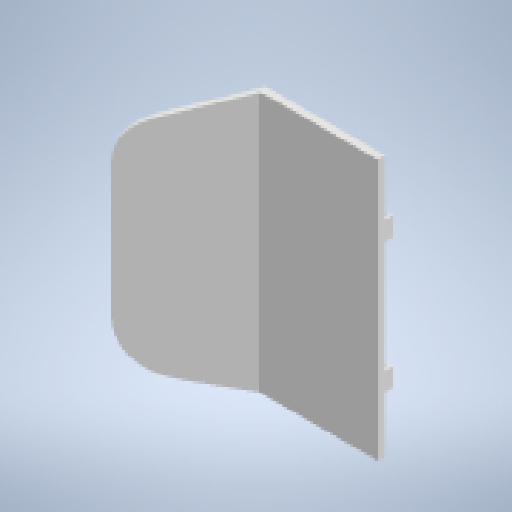
# Autodesk Inventor part: case
Saved by Autodesk Inventor 2025 (Build 290162000, 162)
## iProperties
Created: 2025-08-16
Part Number: case
Material: Generic
Document SubType Name: Modeling
Designer: naka6
Density: 1 g/cm^3
Appearance: Default
Author: naka6
Autodesk Inventor part; units mm, degrees
ref_plane "YZ Plane" through (0, 0, 0) normal (1, 0, 0) x (0, 1, 0)
ref_plane "XZ Plane" through (0, 0, 0) normal (0, 1, 0) x (-1, 0, 0)
ref_plane "XY Plane" through (0, 0, 0) normal (0, 0, 1) x (1, 0, 0)
sketch "スケッチ1" plane through (0, 0, 0) normal (0, 0, 1) x (1, 0, 0)
  line L0 (0, 0) -> (-32, 0)
  line L1 (-32, 0) -> (-32, -70)
  line L2 (-32, -70) -> (0, -70)
  line L3 (0, -70) -> (0, 0)
  dimension "d0" = 32
  dimension "d1" = 70
  constraints: 8 end point, 2 parallel, 1 horizontal, 1 perpendicular
  measures "d0" distance of L0.start L0.end
  measures "d1" distance of L2.end L0.start
extrude "押し出し1" add sketch "スケッチ1" along normal blind 2
sketch "スケッチ2" plane through (-32, -70, 0) normal (0, -1, 0) x (1, 0, 0)
  line L0 (0, 0) -> (32, 0) projected
  line L1 (32, 0) -> (32, 2) projected
  line L2 (0, 2) -> (32, 2) projected
  line L3 (0, 0) -> (0, 2) projected
  line L4 (0, 0) -> (-25.9808, 15)
  line L5 (-25.9808, 15) -> (-25.1147, 16.5)
  line L6 (-25.1147, 16.5) -> (0, 2)
  point P0 (32, 0)
  dimension "d4" = 30
  dimension "d5" = 150
  constraints: 6 end point, 2 perpendicular
  measures "d4" distance of L0.start L4.end
  measures "d5" angle of L2 L6
extrude "押し出し2" add sketch "スケッチ2" against normal blind 70 contours L4 L5 L6 L3
sketch "スケッチ3" plane through (0, 0, 0) normal (0, 0, -1) x (-1, 0, 0)
  line L0 (0, 0) -> (32, 0) projected
  line L1 (32, 0) -> (57.9808, -12.115)
  line L2 (32, 0) -> (57.9808, 0) projected
  line L3 (57.9808, -70) -> (57.9808, 0) projected
  dimension "d8" = 25
  constraints: 2 end point, 1 point on line
  measures "d8" angle of L2 L1
extrude "押し出し3" cut sketch "スケッチ3" against normal blind 70
sketch "スケッチ4" plane through (0, 0, 0) normal (0, 0, -1) x (-1, 0, 0)
  circle A0 centre (9.1, -14.36) radius 1.15 projected
  circle A1 centre (29.46, -53.14) radius 1.15 projected
  circle A2 centre (9.1, -14.36) radius 1
  circle A3 centre (29.46, -53.14) radius 1
  point P0 (0, 0)
  dimension "d11" = 2
  dimension "d12" = 2
  constraints: 2 centre point, 2 coincident
  measures "d11" diameter of A2
  measures "d12" diameter of A3
extrude "押し出し4" add sketch "スケッチ4" along normal blind 5 contours A2 | A3
sketch "スケッチ5" plane through (0, 0, 0) normal (0, 0, -1) x (-1, 0, 0)
  circle A0 centre (9.1, -14.36) radius 1 projected
  circle A1 centre (29.46, -53.14) radius 1 projected
  circle A2 centre (9.1, -14.36) radius 2
  circle A3 centre (29.46, -53.14) radius 2
  line L0 (9.1, -14.36) -> (29.46, -14.36)
  line L1 (29.46, -14.36) -> (29.46, -53.14)
  line L2 (29.46, -53.14) -> (9.1, -53.14)
  line L3 (9.1, -53.14) -> (9.1, -14.36)
  circle A4 centre (29.46, -14.36) radius 2
  circle A5 centre (9.1, -53.14) radius 2
  point P0 (0, 0)
  dimension "d15" = 4
  dimension "d16" = 4
  dimension "d17" = 4
  dimension "d18" = 4
  constraints: 8 end point, 4 centre point, 4 coincident, 2 parallel, 1 horizontal, 1 perpendicular
  measures "d15" diameter of A2
  measures "d16" diameter of A3
  measures "d17" diameter of A4
  measures "d18" diameter of A5
extrude "押し出し5" add sketch "スケッチ5" along normal blind 2 contours L0 L3 A0 | L0 A2 L3 A0 | A0 L3 L0 | A0 L3 A2 L0 | A4 L1 L0 | L0 L1 A4 | A5 L2 L3 | L3 L2 A5 | L1 A1 L2 A3 | A3 L2 A1 L1
sketch "スケッチ6" plane through (-32, -70, 0) normal (-0.5, 0, -0.8660254) x (-0.8660254, 0, 0.5)
  circle A0 centre (6, 56) radius 4 projected
  line L0 (12, 62) -> (0, 62) projected
  line L1 (0, 62) -> (0, 50) projected
  line L2 (0, 50) -> (12, 50) projected
  line L3 (12, 50) -> (12, 62) projected
  line L4 (12.5, 62.5) -> (-0.5, 62.5)
  line L5 (-0.5, 62.5) -> (-0.5, 49.5)
  line L6 (-0.5, 49.5) -> (12.5, 49.5)
  line L7 (12.5, 49.5) -> (12.5, 62.5)
  line L8 (13.5, 63.5) -> (-1.5, 63.5)
  line L9 (-1.5, 63.5) -> (-1.5, 48.5)
  line L10 (-1.5, 48.5) -> (13.5, 48.5)
  line L11 (13.5, 48.5) -> (13.5, 63.5)
  line L12 (4, 48.5) -> (8, 48.5)
  line L13 (8, 48.5) -> (8, 49.5)
  line L14 (8, 49.5) -> (4, 49.5)
  line L15 (4, 49.5) -> (4, 48.5)
  line L16 (4, 62.5) -> (8, 62.5)
  line L17 (8, 62.5) -> (8, 63.5)
  line L18 (8, 63.5) -> (4, 63.5)
  line L19 (4, 63.5) -> (4, 62.5)
  line L20 (6, 48.5) -> (6, 63.5)
  line L21 (0, 70) -> (0, 0) projected
  line L22 (0, 48.5) -> (0, 63.5)
  line L23 (12.5, 57.5369) -> (13.5, 57.5369)
  point P0 (-27.7128, 70)
  point P1 (0, 62.5)
  point P2 (0, 49.5)
  point P3 (4, 49.5)
  dimension "d21" = 0.5
  dimension "d22" = 1
  dimension "d23" = 4
  dimension "d24" = 7.5
  dimension "d25" = 2
  constraints: 38 end point, 12 point on line, 4 parallel, 4 perpendicular, 2 horizontal, 2 midpoint, 6 other
  measures "d21" distance between parallel lines of L3 L7
  measures "d22" distance between parallel lines of L7 L11
  measures "d23" distance between parallel lines of L13 L15
  measures "d24" distance between parallel lines of L11 L20
  measures "d25" distance between parallel lines of L20 L13
extrude "押し出し6" add sketch "スケッチ6" along normal blind 3 contours L21 L8 L19 L4 | L6 L15 L10 L21 | L6 L7 L23 L11 L10 L13
sketch "スケッチ9" plane through (-57.9808, -70, 15) normal (-0.5, 0, -0.8660254) x (-0.8660254, 0, 0.5)
  line L0 (-57.7128, 70) -> (-30, 70) projected
  spline S0 degree 3 poles (-17.6456, 0) (-14.5389, 0) (-12.4319, 0.0723) (-9.2674, 0.5484) (-7.4551, 0.9854) (-4.3314, 2.8768) (-3.1964, 3.9013) (-1.5196, 6.1498) (-0.9279, 7.3003) (-0.1818, 9.6493) (0, 10.8209) (0, 12) knots 0 0 0 0 0.932002 0.932002 1.694801 1.694801 2.239825 2.239825 2.701159 2.701159 3.124298 3.124298 3.124298 3.124298 projected
  spline S1 degree 3 poles (0, 48.1402) (0, 49.6683) (-0.3054, 51.1785) (-1.3061, 53.5747) (-2.0656, 55.0439) (-4.46, 57.4051) (-5.4298, 58.109) (-8.0471, 59.7175) (-9.9104, 60.6321) (-11.1228, 61.1974) knots 0 0 0 0 0.458444 0.458444 0.77844 0.77844 0.966355 0.966355 1.242442 1.242442 1.242442 1.242442 projected
  line L1 (-11.1228, 61.1974) -> (-28.9954, 69.5315) projected
  line L2 (-11.1228, 61.1974) -> (-28.9954, 69.5315) projected
  arc A0 (-28.9954, 69.5315) -> (-31.1085, 70) centre (-31.1085, 65) ccw projected
  line L3 (0, 57.885) -> (-30, 70) projected
  line L4 (0, 0) -> (0, 57.885) projected
  line L5 (0, 0) -> (-30, 0) projected
  line L6 (0, 57.885) -> (0, 70)
  line L7 (0, 70) -> (-31.1085, 70)
  point P0 (-53.3827, 70)
  point P1 (-30, 70)
  constraints: 4 end point, 1 perpendicular, 1 vertical
extrude "押し出し9" cut sketch "スケッチ9" against normal blind 70
sketch "スケッチ10" plane through (-32, -70, 0) normal (-0.5, 0, -0.8660254) x (-0.8660254, 0, 0.5)
  spline S0 degree 3 poles (12.3544, 2) (14.3729, 2) (16.0097, 2.0362) (19.2589, 2.3162) (21.0143, 2.657) (23.8072, 4.1137) (24.8109, 4.9066) (26.4147, 6.7969) (27.0131, 7.8518) (27.7245, 9.9614) (27.8914, 10.977) (27.8914, 11.9999) knots 0 0 0 0 0.605548 0.605548 1.419175 1.419175 1.976207 1.976207 2.502247 2.502247 2.949437 2.949437 2.949437 2.949437 projected
  spline S1 degree 3 poles (27.8914, 48.1552) (27.8914, 49.4139) (27.6391, 50.6569) (26.7879, 52.6951) (26.1446, 53.898) (24.1844, 55.8315) (23.3911, 56.4221) (21.0683, 57.9103) (19.2685, 58.8082) (18.0319, 59.3848) knots 0 0 0 0 0.377607 0.377607 0.661941 0.661941 0.825328 0.825328 1.114005 1.114005 1.114005 1.114005 projected
  line L0 (27.8981, 15.078) -> (26.2914, 15.078)
  line L1 (26.2914, 15.078) -> (26.2914, 20.078)
  line L2 (26.2914, 20.078) -> (27.8981, 20.078)
  line L3 (27.8981, 20.078) -> (27.8981, 15.078)
  line L4 (27.8981, 15.078) -> (27.9914, 15.078)
  line L5 (27.9914, 15.078) -> (27.9914, 20.078)
  line L6 (27.9914, 20.078) -> (27.8981, 20.078)
  line L7 (27.8981, 20.078) -> (27.8981, 15.078)
  spline S2 degree 3 poles (12.3544, 2) (14.3729, 2) (16.0097, 2.0362) (19.2589, 2.3162) (21.0143, 2.657) (23.8072, 4.1137) (24.8109, 4.9066) (26.4147, 6.7969) (27.0131, 7.8518) (27.7245, 9.9614) (27.8914, 10.977) (27.8914, 11.9999) knots 0 0 0 0 0.605548 0.605548 1.419175 1.419175 1.976207 1.976207 2.502247 2.502247 2.949437 2.949437 2.949437 2.949437 projected
  spline S3 degree 3 poles (27.8914, 48.1552) (27.8914, 49.4139) (27.6391, 50.6569) (26.7879, 52.6951) (26.1446, 53.898) (24.1844, 55.8315) (23.3911, 56.4221) (21.0683, 57.9103) (19.2685, 58.8082) (18.0319, 59.3848) knots 0 0 0 0 0.377607 0.377607 0.661941 0.661941 0.825328 0.825328 1.114005 1.114005 1.114005 1.114005 projected
  line L8 (30, 12) -> (30, 48.1402) projected
  line L9 (27.9457, 30.078) -> (29.9457, 30.078)
  line L10 (27.8981, 45.078) -> (26.2914, 45.078)
  line L11 (26.2914, 45.078) -> (26.2914, 40.078)
  line L12 (26.2914, 40.078) -> (27.8981, 40.078)
  line L13 (27.8981, 40.078) -> (27.8981, 45.078)
  line L14 (27.8981, 45.078) -> (27.9914, 45.078)
  line L15 (27.9914, 45.078) -> (27.9914, 40.078)
  line L16 (27.9914, 40.078) -> (27.8981, 40.078)
  line L17 (27.8981, 40.078) -> (27.8981, 45.078)
  line L18 (27.8914, 22.078) -> (27.8914, 38.078) projected
  point P0 (-27.7128, 70)
  point P1 (30, 48.1402)
  point P2 (28.9457, 30.078)
  point P3 (27.0948, 15.078)
  point P4 (27.0948, 45.078)
  point P5 (27.8981, 40.078)
  dimension "d34" = 5
  dimension "d38" = 5
  dimension "d55" = 15
  dimension "d58" = 0.1
  dimension "d59" = 1.6
  dimension "d60" = 8
  dimension "d61" = 2
  constraints: 34 end point, 8 symmetric about line, 4 parallel, 2 horizontal, 2 midpoint, 2 perpendicular, 2 other
  measures "d34" distance of L0.end L1.end
  measures "d38" distance of L4.end L5.end
  measures "d55" vertical distance of point (28.946, 30.078) point (27.095, 15.078)
  measures "d60" distance from line of point (27.891, 22.078) L9
  measures "d61" distance of L9.start L9.end
extrude "押し出し10" add sketch "スケッチ10" along normal blind 3
sketch "スケッチ11" plane through (0, 0, 0) normal (0, 0, -1) x (-1, 0, 0)
  line L0 (0, 0) -> (0, -64.8508)
  line L1 (0, -20) -> (0.9, -20)
  line L2 (0.9, -20) -> (0.9, -15)
  line L3 (0.9, -15) -> (0, -15)
  line L4 (0, -15) -> (0, -20)
  line L5 (0, -35) -> (4.5878, -35)
  line L6 (0, -50) -> (0.9, -50)
  line L7 (0.9, -50) -> (0.9, -55)
  line L8 (0.9, -55) -> (0, -55)
  line L9 (0, -55) -> (0, -50)
  line L10 (0, 0) -> (29.5653, 0) projected
  line L11 (0, -70) -> (0, 0) projected
  point P0 (0, -50)
  point P1 (0, -55)
  point P2 (0, -15)
  dimension "d41" = 5
  dimension "d42" = 15
  dimension "d43" = 0.9
  dimension "d62" = 35
  constraints: 20 end point, 4 symmetric about line, 2 horizontal, 2 parallel, 1 perpendicular, 1 point on line, 1 vertical, 1 other
  measures "d41" distance of L1.end L2.end
  measures "d42" distance from line of L5.start L1
  measures "d43" distance of L1.start L1.end
  measures "d62" distance between parallel lines of L10 L5
extrude "押し出し11" add sketch "スケッチ11" along normal blind 2
sketch "スケッチ12" plane through (-0.9, -55, 0) normal (0, -1, 0) x (1, 0, 0)
  line L0 (0, 0) -> (0.9, 0) projected
  line L1 (0, 0) -> (0, -2) projected
  line L2 (0.9, -2) -> (0, -2) projected
  line L3 (0.9, 0) -> (0.9, -2) projected
  line L4 (0, -2) -> (-0.5, -2)
  line L5 (-0.5, -2) -> (-0.5, -1.5)
  line L6 (-0.5, -1.5) -> (0, -1.5)
  line L7 (0, -1.5) -> (0, -2)
  line L8 (0, -2) -> (-0.5, -1.5)
  point P0 (0.9, 0)
  point P1 (0, -1.5)
  dimension "d46" = 0.5
  dimension "d47" = 0.5
  constraints: 10 end point, 2 parallel, 1 horizontal, 1 perpendicular
  measures "d46" distance of L5.end L6.end
  measures "d47" distance of L4.end L5.end
extrude "押し出し12" add sketch "スケッチ12" against normal blind 5 contours L1 L8 L6
sketch "スケッチ13" plane through (-0.9, -20, 0) normal (0, -1, 0) x (1, 0, 0)
  line L0 (0, 0) -> (0.9, 0) projected
  line L1 (0, 0) -> (0, -1.5) projected
  line L2 (0, -1.5) -> (-0.5, -1.5) projected
  line L3 (-0.5, -1.5) -> (0, -2) projected
  line L4 (0.9, -2) -> (0, -2) projected
  line L5 (0.9, 0) -> (0.9, -2) projected
  line L6 (0, -2) -> (0, -1.5)
  point P0 (0.9, 0)
  constraints: 2 end point, 1 vertical
extrude "押し出し13" add sketch "スケッチ13" against normal blind 5 contours L6 L3 L2
chamfer "面取り1" distance 0.4 angle 45 2 edges at (-0.9, -17.5, 0) (-0.9, -52.5, 0)
